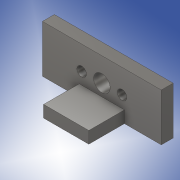
# Autodesk Inventor part: C005
Saved by Autodesk Inventor 2017 (Build 210142000, 142)
## iProperties
Created: 2017-06-13
Part Number: C005
Material: Steel, Carbon
Document SubType Name: Modeling
Designer: zallen
Density: 7.85 g/cm^3
Appearance: Semi-Polished
Mass: 67.5643 g
Surface Area: 46.2838 cm^2
Volume: 8.60691 cm^3
Author: zallen
Autodesk Inventor part; units mm, degrees
ref_plane "YZ Plane" through (0, 0, 0) normal (1, 0, 0) x (0, 1, 0)
ref_plane "XZ Plane" through (0, 0, 0) normal (0, 1, 0) x (-1, 0, 0)
ref_plane "XY Plane" through (0, 0, 0) normal (0, 0, 1) x (1, 0, 0)
sketch "Sketch1" plane through (0, 0, 0) normal (0, 0, 1) x (1, 0, 0)
  line L0 (0, 0) -> (50, 0)
  circle A0 centre (25, 10) radius 3.5
  line L1 (0, 0) -> (0, 20)
  line L2 (0, 20) -> (50, 20)
  line L3 (50, 20) -> (50, 0)
  point P0 (25, 0)
  dimension "d0" = 50
  dimension "d2" = 7
  dimension "d3" = 10
  dimension "d4" = 20
  constraints: 8 end point, 2 perpendicular, 1 centre point, 1 horizontal, 1 midpoint, 1 vertical, 1 vertical alignment
  measures "d0" distance of L0.start L0.end
  measures "d2" diameter of A0
  measures "d3" distance of point (25, 0) A0.centre
  measures "d4" distance of L0.start L1.end
extrude "Extrusion1" add sketch "Sketch1" along normal blind 5
sketch "Sketch2" plane through (0, 0, 5) normal (0, 0, 1) x (1, 0, 0)
  line L0 (0, 0) -> (50, 0) projected
  line L1 (15.5, 0) -> (34.5, 0)
  line L2 (34.5, 0) -> (34.5, 5)
  line L3 (34.5, 5) -> (15.5, 5)
  line L4 (15.5, 5) -> (15.5, 0)
  point P0 (25, 0)
  dimension "d7" = 19
  dimension "d8" = 5
  constraints: 8 end point, 2 midpoint, 2 parallel, 1 horizontal, 1 perpendicular, 1 point on line
  measures "d7" distance of L3.end L2.end
  measures "d8" distance of L1.end L2.end
extrude "Extrusion2" add sketch "Sketch2" along normal blind 15
sketch "Sketch3" plane through (0, 0, 5) normal (0, 0, 1) x (1, 0, 0)
  circle A0 centre (16.5, 10) radius 2
  circle A1 centre (33.5, 10) radius 2
  line L0 (34.5, 5) -> (34.5, 0) projected
  line L1 (34.5, 0) -> (50, 0) projected
  line L2 (50, 0) -> (50, 20) projected
  line L3 (50, 20) -> (0, 20) projected
  line L4 (0, 20) -> (0, 0) projected
  line L5 (0, 0) -> (15.5, 0) projected
  line L6 (15.5, 0) -> (15.5, 5) projected
  line L7 (15.5, 5) -> (34.5, 5) projected
  circle A2 centre (25, 10) radius 3.5 projected
  line L8 (16.5, 10) -> (33.5, 10) construction
  dimension "d11" = 4
  dimension "d12" = 4
  dimension "d13" = 17
  constraints: 2 centre point, 2 end point, 1 coincident, 1 horizontal, 1 horizontal alignment, 1 midpoint
  measures "d11" diameter of A0
  measures "d12" diameter of A1
  measures "d13" distance of L8.end L8.start
extrude "Extrusion3" cut sketch "Sketch3" against normal through all contours A0 | A1
body "Solid1"
